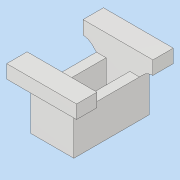
# Autodesk Inventor part: ForeConnectorHolder
Saved by Autodesk Inventor 2017 (Build 210142000, 142)
## iProperties
Created: 2019-07-13
Part Number: ForeConnectorHolder
Material: ABS Plastic
Document SubType Name: Modeling
Designer: techn
Density: 1.06 g/cm^3
Appearance: Smooth - White
Author: techn
Autodesk Inventor part; units mm, degrees
ref_plane "YZ Plane" through (0, 0, 0) normal (1, 0, 0) x (0, 1, 0)
ref_plane "XZ Plane" through (0, 0, 0) normal (0, 1, 0) x (-1, 0, 0)
ref_plane "XY Plane" through (0, 0, 0) normal (0, 0, 1) x (1, 0, 0)
sketch "Sketch1" plane through (0, 0, 0) normal (0, 1, 0) x (-1, 0, 0)
  line L0 (0, 0) -> (10.16, 0)
  line L1 (10.16, 0) -> (10.16, -17.78)
  line L2 (10.16, -17.78) -> (0, -17.78)
  line L3 (0, -17.78) -> (0, 0)
  line L4 (7.874, -15.494) -> (7.874, -2.286)
  line L5 (7.874, -2.286) -> (2.286, -2.286)
  line L6 (2.286, -2.286) -> (2.286, -15.494)
  line L7 (2.286, -15.494) -> (7.874, -15.494)
  dimension "d0" = 17.78
  dimension "d1" = 10.16
  dimension "d2" = 2.286
  constraints: 16 end point, 4 parallel, 2 perpendicular, 1 horizontal, 3 other
  measures "d0" distance of L2.end L0.start
  measures "d1" distance of L1.end L2.end
  measures "d2" distance between parallel lines of L1 L4
extrude "Extrusion1" add sketch "Sketch1" along normal blind 8.89
sketch "Sketch2" plane through (0, 8.89, 0) normal (0, 1, 0) x (1, 0, 0)
  line L0 (-10.16, 0) -> (0, 0) projected
  line L1 (-2.286, 2.286) -> (-7.874, 2.286) projected
  line L2 (-7.874, 15.494) -> (-2.286, 15.494) projected
  line L3 (0, 17.78) -> (-10.16, 17.78) projected
  line L4 (-10.16, 0) -> (0, 0)
  line L5 (0, 0) -> (0, 2.286)
  line L6 (0, 2.286) -> (-10.16, 2.286)
  line L7 (-10.16, 2.286) -> (-10.16, 0)
  line L8 (-10.16, 0) -> (-10.16, 17.78) projected
  line L9 (0, 17.78) -> (-10.16, 17.78)
  line L10 (-10.16, 17.78) -> (-10.16, 15.494)
  line L11 (-10.16, 15.494) -> (0, 15.494)
  line L12 (0, 15.494) -> (0, 17.78)
  constraints: 16 end point, 4 parallel, 2 horizontal, 2 perpendicular, 1 point on line
extrude "Extrusion2" add sketch "Sketch2" along normal blind 5.08
sketch "Sketch3" plane through (0, 13.97, 0) normal (0, 1, 0) x (1, 0, 0)
  line L0 (-10.16, 0) -> (0, 0) projected
  line L1 (0, 17.78) -> (-10.16, 17.78) projected
  line L2 (-10.16, 15.494) -> (0, 15.494) projected
  line L3 (0, 15.494) -> (0, 17.78) projected
  line L4 (0, 17.78) -> (-10.16, 17.78) projected
  line L5 (-10.16, 17.78) -> (-10.16, 15.494) projected
  line L6 (-10.16, 0) -> (0, 0) projected
  line L7 (0, 0) -> (0, 2.286) projected
  line L8 (0, 2.286) -> (-10.16, 2.286) projected
  line L9 (-10.16, 2.286) -> (-10.16, 0) projected
  line L10 (-13.335, 2.286) -> (3.175, 2.286)
  line L11 (3.175, 2.286) -> (3.175, -2.54)
  line L12 (3.175, -2.54) -> (-13.335, -2.54)
  line L13 (-13.335, -2.54) -> (-13.335, 2.286)
  line L14 (-13.335, 15.494) -> (3.175, 15.494)
  line L15 (3.175, 15.494) -> (3.175, 20.32)
  line L16 (3.175, 20.32) -> (-13.335, 20.32)
  line L17 (-13.335, 20.32) -> (-13.335, 15.494)
  dimension "d7" = 3.175
  dimension "d8" = 3.175
  dimension "d9" = 2.54
  dimension "d10" = 2.54
  constraints: 16 end point, 4 parallel, 2 horizontal, 2 perpendicular, 2 point on line
  measures "d7" distance between parallel lines of L13 L9
  measures "d8" distance between parallel lines of L7 L11
  measures "d9" distance between parallel lines of L0 L12
  measures "d10" distance between parallel lines of L16 L1
extrude "Extrusion3" add sketch "Sketch3" against normal blind 3.175 contours L0 L7 L10 L11 L12 L13 L9 | L1 L5 L14 L17 L16 L15 L3
chamfer "Chamfer1" distance 1.905 angle 45 6 edges at (-5.08, 10.795, 0) (0, 10.795, -1.143) (-10.16, 10.795, -1.143) (0, 10.795, -16.637) (-5.08, 10.795, -17.78) (-10.16, 10.795, -16.637)
fillet "Fillet1" radius 3.175 6 edges at (1.905, 10.795, -17.5895) (-5.08, 10.795, -19.685) (-12.065, 10.795, -17.5895) (-12.065, 10.795, -0.1905) (-5.08, 10.795, 1.905) (1.905, 10.795, -0.1905)
body "Solid1"
